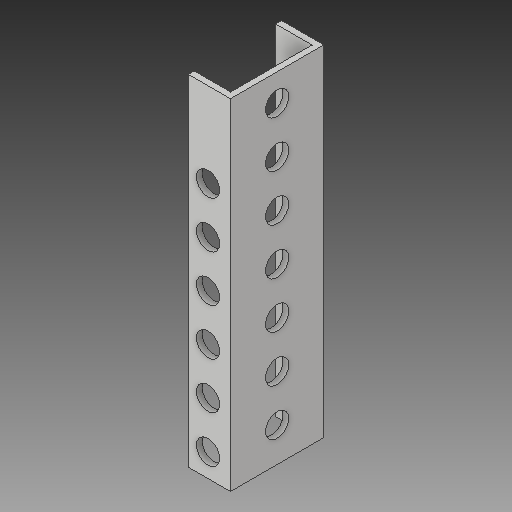
# Autodesk Inventor part: Base C Channel
Saved by Autodesk Inventor 2018 (Build 220112000, 112)
## iProperties
Created: 2017-06-28
Part Number: Base C Channel
Material: Generic
Document SubType Name: Sheet Metal
Designer: James
Density: 1 g/cm^3
Appearance: Default
Sheet Metal Rule: Default_mm
Mass: 5.76937 g
Surface Area: 82.9046 cm^2
Volume: 5.76937 cm^3
Author: James
Autodesk Inventor part; units mm, degrees
ref_plane "YZ Plane" through (0, 0, 0) normal (1, 0, 0) x (0, 1, 0)
ref_plane "XZ Plane" through (0, 0, 0) normal (0, 1, 0) x (-1, 0, 0)
ref_plane "XY Plane" through (0, 0, 0) normal (0, 0, 1) x (1, 0, 0)
sketch "Sketch1" plane through (0, 0, 0) normal (0, 1, 0) x (-1, 0, 0)
  line L0 (8.9296, 2.0793) -> (8.9296, 0.4537)
  line L1 (8.9296, 0.4537) -> (-1.0304, 0.4537)
  line L2 (8.9296, 2.0793) -> (-1.0304, 2.0793)
  line L3 (-1.0304, 0.4537) -> (-1.0304, -21.7963)
  line L4 (-1.0304, -21.7963) -> (8.9312, -21.7963)
  line L5 (8.9312, -21.7963) -> (8.9312, -23.4219)
  line L6 (8.9312, -23.4219) -> (-2.6004, -23.4219)
  line L7 (-2.6004, 2.0793) -> (-1.0304, 2.0793)
  line L8 (-2.6004, 2.0793) -> (-2.6004, -23.4219)
  dimension "d1" = 1.6256
  dimension "d2" = 22.25
  dimension "d3" = 1.6256
  dimension "d4" = 1.57
  dimension "d5" = 9.96
  dimension "d6" = 1.57
  dimension "d7" = 11.5316
  constraints: 18 end point, 3 perpendicular, 3 vertical, 2 horizontal
  measures "d1" distance between parallel lines of L1 L2
  measures "d2" distance of L1.end L3.end
  measures "d3" distance between parallel lines of L4 L6
  measures "d4" distance between parallel lines of L3 L8
  measures "d5" distance of L0.start L2.end
  measures "d6" distance of L7.start L2.end
  measures "d7" distance of L5.end L6.end
extrude "Extrusion1" add sketch "Sketch1" along normal blind 93
sketch "Sketch2" plane through (1.0304, 0, -21.7963) normal (-1, 0, 0) x (0, 0, 1)
  line L0 (22.25, 0) -> (22.25, 93) projected
  line L1 (0, 0) -> (0, 93) projected
  circle A0 centre (11.1238, 9.3725) radius 2.1468
  line L2 (22.25, 0) -> (0, 0) projected
  circle A1 centre (11.125, 22.0725) radius 2.1468
  circle A2 centre (11.125, 34.7725) radius 2.1468
  circle A3 centre (11.125, 47.4725) radius 2.1468
  circle A4 centre (11.125, 60.1725) radius 2.1468
  circle A5 centre (11.125, 72.8725) radius 2.1468
  circle A6 centre (11.125, 85.5725) radius 2.1468
  point P0 (21.7963, 0)
  dimension "d14" = 11.1262
  dimension "d15" = 9.3725
  dimension "d23" = 4.2935
  dimension "d24" = 4.2935
  dimension "d25" = 11.125
  dimension "d26" = 12.7
  dimension "d27" = 4.2935
  dimension "d28" = 12.7
  dimension "d29" = 4.2935
  dimension "d30" = 12.7
  dimension "d31" = 4.2935
  dimension "d32" = 12.7
  dimension "d33" = 4.2935
  dimension "d34" = 12.7
  dimension "d35" = 4.2935
  dimension "d36" = 12.7
  constraints: 7 centre point
  measures "d14" distance from line of L0 A0.centre
  measures "d15" distance from line of L2 A0.centre
  measures "d23" diameter of A0
  measures "d24" diameter of A1
  measures "d25" distance from line of L0 A1.centre
  measures "d26" distance of A0.centre A1.centre
  measures "d27" diameter of A2
  measures "d28" distance of A1.centre A2.centre
  measures "d29" diameter of A3
  measures "d30" distance of A2.centre A3.centre
  measures "d31" diameter of A4
  measures "d32" distance of A3.centre A4.centre
  measures "d33" diameter of A5
  measures "d34" distance of A4.centre A5.centre
  measures "d35" diameter of A6
  measures "d36" distance of A5.centre A6.centre
hole "Hole3" at (1.0304, 9.3725, -10.6725) at (1.0304, 22.0725, -10.6713) at (1.0304, 34.7725, -10.6713) at (1.0304, 47.4725, -10.6713) at (1.0304, 60.1725, -10.6713) at (1.0304, 72.8725, -10.6713) at (1.0304, 85.5725, -10.6713) direction (1, 0, 0) diameter 6.35 end through all
sketch "Sketch3" plane through (-8.9296, 0, 2.0793) normal (0, 0, 1) x (1, 0, 0)
  line L0 (11.53, 0) -> (0, 0) projected
  line L1 (11.53, 0) -> (11.53, 93) projected
  circle A0 centre (5.3929, 6.35) radius 2.3114
  line L2 (0, 0) -> (0, 93) projected
  circle A1 centre (5.3929, 19.05) radius 2.3114
  circle A2 centre (5.3929, 31.75) radius 2.3114
  circle A3 centre (5.3929, 44.45) radius 2.3114
  circle A4 centre (5.3929, 57.15) radius 2.3114
  circle A5 centre (5.3929, 69.85) radius 2.3114
  point P0 (8.9296, 0)
  dimension "d55" = 6.35
  dimension "d56" = 4.6228
  dimension "d57" = 5.3929
  dimension "d58" = 4.6228
  dimension "d59" = 12.7
  dimension "d60" = 4.6228
  dimension "d61" = 12.7
  dimension "d62" = 4.6228
  dimension "d63" = 12.7
  dimension "d64" = 4.6228
  dimension "d65" = 12.7
  dimension "d66" = 4.6228
  dimension "d67" = 12.7
  constraints: 6 centre point
  measures "d55" distance from line of L0 A0.centre
  measures "d56" diameter of A0
  measures "d57" distance from line of L2 A0.centre
  measures "d58" diameter of A1
  measures "d59" distance of A0.centre A1.centre
  measures "d60" diameter of A2
  measures "d61" distance of A1.centre A2.centre
  measures "d62" diameter of A3
  measures "d63" distance of A2.centre A3.centre
  measures "d64" diameter of A4
  measures "d65" distance of A3.centre A4.centre
  measures "d66" diameter of A5
  measures "d67" distance of A4.centre A5.centre
hole "Hole4" at (-3.5367, 69.85, 2.0793) at (-3.5367, 57.15, 2.0793) at (-3.5367, 44.45, 2.0793) at (-3.5367, 31.75, 2.0793) at (-3.5367, 19.05, 2.0793) at (-3.5367, 6.35, 2.0793) direction (0, 0, -1) diameter 6.35 end through all
equation "\"d49\" = Thickness"
equation "\"d73\" = Thickness"
equation "\"BendRadius\" = Thickness"
equation "\"BendReliefWidth\" = Thickness"
equation "\"BendReliefDepth\" = 0.5 * Thickness"
equation "\"CornerReliefSize\" = 4 * Thickness"
equation "\"MinimumRemnant\" = 2 * Thickness"
equation "\"TransitionRadius\" = BendRadius"
equation "\"JacobiRadiusSize\" = BendRadius"
equation "\"GapSize\" = Thickness"
equation "\"Thickness\" = 1.6256"
body "Solid1"
